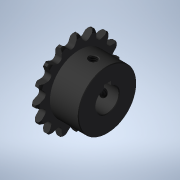
# Autodesk Inventor part: FBN25B16D10_()
Saved by Autodesk Inventor 2021 (Build 250183000, 183)
## iProperties
Created: 2025-03-16
Part Number: FBN25B16D10_()
Material: Generic
Catalog Web Link: www.cadenas.de
Description: FBN25B-Finished bore
Vendor: KANA
Document SubType Name: Modeling
Designer: psAdmin
Manufacturer: KANA
Mass: 6.8832 g
Surface Area: 34.2887 cm^2
Volume: 6.8832 cm^3
Density: 1 g/cm^3
Appearance: PSOLRGB-175-175-175
Category: PARTsolutions
Company: KANA
Title: FBN25B16D10
Author: Cadenas PARTsolutions
Comments: Finished bore
PSOL_IDENT_0: {$CADENAS_DATA/23d-libs/kana/sprockets/chain_no_25/finished_bore_sprocket_steel_stainless/b_type/fbn
PSOL_IDENT_1: 25b.prj},178 {VTYP=3D},{NB=FBN25B16D10_()},{LINA=FBN25B16D10},{NN=FBN25B},{DATE=07.03.2025 00:51:18}
PSOL_IDENT_2: ,{GEOMDATE=02.10.2020 05:05:34},{VERSION=},{LINEID=10},{WBVAR=SD,KS,SURFT},{WBNUMERIC=SD}  {NB=FBN25
PSOL_IDENT_3: B16D10_()},{LINA=FBN25B16D10},{KT=DUMMY},{ORDERNO=FBN25B16D10},{TYPE=FBN25B},{NOT=16},{NOTX=16.000},
PSOL_IDENT_4: {DP=32.55},{DO=36},{DC=29.25},{DC2=29.25},{T=2.8},{DR=3.3},{MAT=None},{MATC=},{SHAPE=C : Cutting typ
PSOL_IDENT_5: e},{SHAPENB=C},{SD=10},{SDX=10,12},{KS=3 X 1.4},{KSX='3 X 1.4','4 X 1.8'},{M=M4},{NOTHP=2},{A=6},{SU
PSOL_IDENT_6: RFT=},{SURFTNB=},{BD=25},{BL=15},{GD=0},{GDX=0},{S=0},{X=0},{VS=0},{SVDEL1=12},{SVDEL4=4},{SVDEL5=52
PSOL_IDENT_7: },{DCX2=0},{B=3},{T2=1.4},{ANGLE=0},{NDM=4},{KDM=3.242},{ONX=},{CAUTION=The tooth profile in the CAD
PSOL_IDENT_8: models differ from the actual shape.}
NB: FBN25B16D10_()
NN: FBN25B
NT: Finished bore
NBSYN: FBN25B$NOT.D$SD.$ONX._($SURFT.)
LINA: FBN25B16D10
CATALOG: KANA
TYPE: FBN25B
NOT: 16
DP: 32.55
DO: 36
DC: 29.25
DC2: 29.25
T: 2.8
SHAPE: C : Cutting type
SD: 10
KS: 3 X 1.4
M: M4
NOTHP: 2
A: 6
SURFT: No symbol : No
CAUTION: The tooth profile in the CAD models differ from the actual shape.
SUPPLIER: KANA
ARTICLENO: FBN25B16D10_()
BOMINFO: FBN25B16D10
CREATOR: CADENAS GmbH
Autodesk Inventor part; units mm, degrees
ref_plane "YZ Plane" through (0, 0, 0) normal (1, 0, 0) x (0, 1, 0)
ref_plane "XZ Plane" through (0, 0, 0) normal (0, 1, 0) x (-1, 0, 0)
ref_plane "XY Plane" through (0, 0, 0) normal (0, 0, 1) x (1, 0, 0)
sketch "Sketch_1" plane through (0, 0, 0) normal (0, 0, 1) x (1, 0, 0)
  line L0 (15, 0) -> (0, 0)
  line L1 (0, 5.25) -> (0.25, 5)
  line L2 (0.25, 5) -> (14.75, 5)
  line L3 (14.75, 5) -> (15, 5.25)
  line L4 (15, 5.25) -> (15, 12.25)
  line L5 (15, 12.25) -> (14.75, 12.5)
  line L6 (14.75, 12.5) -> (2.8, 12.5)
  line L7 (2.8, 12.5) -> (2.8, 16.8899)
  arc A0 (2.8, 16.8899) -> (2.1, 18) centre (-0.2857, 15.7199) ccw
  line L8 (2.1, 18) -> (0.7, 18)
  arc A1 (0.7, 18) -> (0, 16.8899) centre (3.0857, 15.7199) ccw
  line L9 (0, 16.8899) -> (0, 5.25)
  constraints: 20 end point, 4 point on circle, 2 centre point
revolve "Revolution1" add sketch "Sketch_1" angle 360 about axis through (15, 0, 0) along (1, 0, 0)
sketch "Sketch_7" plane through (1.4, 0, 0) normal (1, 0, 0) x (0, 0, -1)
  circle A0 centre (0, 0) radius 24
  arc A1 (-17.9931, 0.5) -> (-17.9931, -0.5) centre (0, 0) ccw
  line L0 (-17.9931, -0.5) -> (-15.3077, -1.6605)
  arc A2 (-14.7779, -4.3239) -> (-15.3077, -1.6605) centre (-15.9623, -3.1751) ccw
  line L1 (-14.7779, -4.3239) -> (-16.8148, -6.4237)
  arc A3 (-16.8148, -6.4237) -> (-16.4321, -7.3476) centre (0, 0) ccw
  line L2 (-16.4321, -7.3476) -> (-13.5071, -7.3921)
  arc A4 (-11.9983, -9.6501) -> (-13.5071, -7.3921) centre (-13.5322, -9.0419) ccw
  line L3 (-11.9983, -9.6501) -> (-13.0766, -12.3695)
  arc A5 (-13.0766, -12.3695) -> (-12.3695, -13.0766) centre (0, 0) ccw
  line L4 (-12.3695, -13.0766) -> (-9.6501, -11.9983)
  arc A6 (-7.3921, -13.5071) -> (-9.6501, -11.9983) centre (-9.0419, -13.5322) ccw
  line L5 (-7.3921, -13.5071) -> (-7.3476, -16.4321)
  arc A7 (-7.3476, -16.4321) -> (-6.4237, -16.8148) centre (0, 0) ccw
  line L6 (-6.4237, -16.8148) -> (-4.3239, -14.7779)
  arc A8 (-1.6605, -15.3077) -> (-4.3239, -14.7779) centre (-3.1751, -15.9623) ccw
  line L7 (-1.6605, -15.3077) -> (-0.5, -17.9931)
  arc A9 (-0.5, -17.9931) -> (0.5, -17.9931) centre (0, 0) ccw
  line L8 (0.5, -17.9931) -> (1.6605, -15.3077)
  arc A10 (4.3239, -14.7779) -> (1.6605, -15.3077) centre (3.1751, -15.9623) ccw
  line L9 (4.3239, -14.7779) -> (6.4237, -16.8148)
  arc A11 (6.4237, -16.8148) -> (7.3476, -16.4321) centre (0, 0) ccw
  line L10 (7.3476, -16.4321) -> (7.3921, -13.5071)
  arc A12 (9.6501, -11.9983) -> (7.3921, -13.5071) centre (9.0419, -13.5322) ccw
  line L11 (9.6501, -11.9983) -> (12.3695, -13.0766)
  arc A13 (12.3695, -13.0766) -> (13.0766, -12.3695) centre (0, 0) ccw
  line L12 (13.0766, -12.3695) -> (11.9983, -9.6501)
  arc A14 (13.5071, -7.3921) -> (11.9983, -9.6501) centre (13.5322, -9.0419) ccw
  line L13 (13.5071, -7.3921) -> (16.4321, -7.3476)
  arc A15 (16.4321, -7.3476) -> (16.8148, -6.4237) centre (0, 0) ccw
  line L14 (16.8148, -6.4237) -> (14.7779, -4.3239)
  arc A16 (15.3077, -1.6605) -> (14.7779, -4.3239) centre (15.9623, -3.1751) ccw
  line L15 (15.3077, -1.6605) -> (17.9931, -0.5)
  arc A17 (17.9931, -0.5) -> (17.9931, 0.5) centre (0, 0) ccw
  line L16 (17.9931, 0.5) -> (15.3077, 1.6605)
  arc A18 (14.7779, 4.3239) -> (15.3077, 1.6605) centre (15.9623, 3.1751) ccw
  line L17 (14.7779, 4.3239) -> (16.8148, 6.4237)
  arc A19 (16.8148, 6.4237) -> (16.4321, 7.3476) centre (0, 0) ccw
  line L18 (16.4321, 7.3476) -> (13.5071, 7.3921)
  arc A20 (11.9983, 9.6501) -> (13.5071, 7.3921) centre (13.5322, 9.0419) ccw
  line L19 (11.9983, 9.6501) -> (13.0766, 12.3695)
  arc A21 (13.0766, 12.3695) -> (12.3695, 13.0766) centre (0, 0) ccw
  line L20 (12.3695, 13.0766) -> (9.6501, 11.9983)
  arc A22 (7.3921, 13.5071) -> (9.6501, 11.9983) centre (9.0419, 13.5322) ccw
  line L21 (7.3921, 13.5071) -> (7.3476, 16.4321)
  arc A23 (7.3476, 16.4321) -> (6.4237, 16.8148) centre (0, 0) ccw
  line L22 (6.4237, 16.8148) -> (4.3239, 14.7779)
  arc A24 (1.6605, 15.3077) -> (4.3239, 14.7779) centre (3.1751, 15.9623) ccw
  line L23 (1.6605, 15.3077) -> (0.5, 17.9931)
  arc A25 (0.5, 17.9931) -> (-0.5, 17.9931) centre (0, 0) ccw
  line L24 (-0.5, 17.9931) -> (-1.6605, 15.3077)
  arc A26 (-4.3239, 14.7779) -> (-1.6605, 15.3077) centre (-3.1751, 15.9623) ccw
  line L25 (-4.3239, 14.7779) -> (-6.4237, 16.8148)
  arc A27 (-6.4237, 16.8148) -> (-7.3476, 16.4321) centre (0, 0) ccw
  line L26 (-7.3476, 16.4321) -> (-7.3921, 13.5071)
  arc A28 (-9.6501, 11.9983) -> (-7.3921, 13.5071) centre (-9.0419, 13.5322) ccw
  line L27 (-9.6501, 11.9983) -> (-12.3695, 13.0766)
  arc A29 (-12.3695, 13.0766) -> (-13.0766, 12.3695) centre (0, 0) ccw
  line L28 (-13.0766, 12.3695) -> (-11.9983, 9.6501)
  arc A30 (-13.5071, 7.3921) -> (-11.9983, 9.6501) centre (-13.5322, 9.0419) ccw
  line L29 (-13.5071, 7.3921) -> (-16.4321, 7.3476)
  arc A31 (-16.4321, 7.3476) -> (-16.8148, 6.4237) centre (0, 0) ccw
  line L30 (-16.8148, 6.4237) -> (-14.7779, 4.3239)
  arc A32 (-15.3077, 1.6605) -> (-14.7779, 4.3239) centre (-15.9623, 3.1751) ccw
  line L31 (-15.3077, 1.6605) -> (-17.9931, 0.5)
  constraints: 64 end point, 64 point on circle, 33 centre point
extrude "Extrusion1" cut sketch "Sketch_7" along normal mid plane 3.2
sketch "Sketch_2" plane through (0, 0, 0) normal (0, 0, 1) x (1, 0, 0)
  line L0 (9, 0) -> (9, 12.5)
  line L1 (9, 12.5) -> (11, 12.5)
  line L2 (11, 12.5) -> (10.621, 12.121)
  line L3 (10.621, 12.121) -> (10.621, 0)
  line L4 (10.621, 0) -> (9, 0)
  line L5 (9, 0) -> (9, 12.5)
  constraints: 12 end point
revolve "Revolution2" cut sketch "Sketch_2" angle 360 about axis through (9, 0, 0) along (0, -1, 0)
thread "Thread1" size "M4x0.7" class "6H" standard "ISO Metric profile" length 5.721
sketch "Sketch_3" plane through (0, 0, 0) normal (0, 0.8660254, -0.5) x (1, 0, 0)
  line L0 (9, 0) -> (9, 12.5)
  line L1 (9, 12.5) -> (11, 12.5)
  line L2 (11, 12.5) -> (10.621, 12.121)
  line L3 (10.621, 12.121) -> (10.621, 0)
  line L4 (10.621, 0) -> (9, 0)
  line L5 (9, 0) -> (9, 12.5)
  constraints: 12 end point
revolve "Revolution3" cut sketch "Sketch_3" angle 360 about axis through (9, 0, 0) along (0, 0.5, 0.8660254)
thread "Thread2" size "M4x0.7" class "6H" standard "ISO Metric profile" length 5.721
sketch "Sketch_4" plane through (0, 0, 0) normal (1, 0, 0) x (0, 1, 0)
  line L0 (3.6, 1.5) -> (3.6, -1.5)
  line L1 (3.6, -1.5) -> (6.4, -1.5)
  line L2 (6.4, -1.5) -> (6.4, 1.5)
  line L3 (6.4, 1.5) -> (3.6, 1.5)
  constraints: 8 end point
extrude "Extrusion2" cut sketch "Sketch_4" along normal blind 15
ref_plane "body_XY" through (0, 0, 0) normal (1, 0, 0) x (0, 0, -1)
ref_plane "body_YZ" through (0, 0, 0) normal (0, 0, -1) x (0, 1, 0)
ref_plane "body_ZX" through (0, 0, 0) normal (0, 1, 0) x (1, 0, 0)
body "Solid1"
